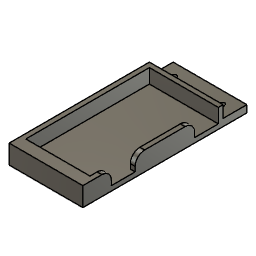
HC-05 mount (Autodesk Fusion 360 design; units mm, degrees)
Autodesk Fusion 360 part; units mm, degrees
sketch "Sketch1" plane through (0, 0, 0) normal (0, 1, 0) x (1, 0, 0)
  line L0 (0, 0) -> (13.5, 0)
  line L1 (13.5, 0) -> (13.5, 27.5)
  line L2 (13.5, 27.5) -> (0, 27.5)
  line L3 (0, 27.5) -> (0, 0)
  dimension "d1" = 13.5
  dimension "d2" = 27.5
  constraint horizontal L0
  constraint vertical L1
  constraint horizontal L2
  constraint vertical L3
  constraint coincident L0.start L3.end
  measures "d1" distance of L0.start L0.end
  measures "d2" distance of L0.start L2.end
extrude "Extrude1" add sketch "Sketch1" along normal blind 1
sketch "Sketch2" plane through (0, 0, 0) normal (0, -1, 0) x (1, 0, 0)
  line L0 (0, 0) -> (0, -27.5)
  line L1 (0, -27.5) -> (13.5, -27.5)
  line L2 (13.5, -27.5) -> (13.5, 0)
  line L3 (13.5, 0) -> (0, 0)
  line L4 (0, -27.5) -> (13.5, -27.5)
  line L5 (13.5, -27.5) -> (13.5, 0)
  line L6 (13.5, 0) -> (0, 0)
  line L7 (0, 0) -> (0, -27.5)
  line L8 (-1, -28.5) -> (14.5, -28.5)
  line L9 (14.5, -28.5) -> (14.5, 1)
  line L10 (14.5, 1) -> (-1, 1)
  line L11 (-1, 1) -> (-1, -28.5)
  dimension "d5" = 1
  constraint horizontal L4
  constraint vertical L5
  constraint horizontal L6
  constraint vertical L7
  constraint coincident L2.end L3.start
  constraint coincident L0.end L1.start
extrude "Extrude2" add sketch "Sketch2" against normal blind 4
sketch "Sketch3" plane through (14.5, 0, 0) normal (1, 0, 0) x (0, 0, -1)
  line L0 (-1, 0) -> (28.5, 0)
  line L1 (28.5, 0) -> (28.5, 4)
  line L2 (28.5, 4) -> (-1, 4)
  line L3 (-1, 4) -> (-1, 0)
  line L4 (28.5, 4) -> (27.5, 4)
  line L5 (27.5, 4) -> (22.5, 4)
  line L6 (22.5, 4) -> (22.5, 1)
  line L7 (22.5, 1) -> (27.5, 1)
  line L8 (27.5, 1) -> (27.5, 4)
  line L9 (-1, 4) -> (5, 4)
  line L10 (5, 4) -> (10, 4)
  line L11 (10, 4) -> (10, 1)
  line L12 (10, 1) -> (5, 1)
  line L13 (5, 1) -> (5, 4)
  dimension "d8" = 5
  dimension "d9" = 6
  dimension "d10" = 5
  dimension "d11" = 3
  constraint coincident L1.end L2.start
  constraint coincident L2 L4.end
  constraint perpendicular L1 L4
  constraint horizontal L5
  constraint vertical L6
  constraint horizontal L7
  constraint vertical L8
  constraint coincident L2.end L3.start
  constraint perpendicular L3 L9
  constraint horizontal L10
  constraint vertical L11
  constraint horizontal L12
  constraint vertical L13
  measures "d8" distance of L4.end L5.end
  measures "d9" distance of L2.end L9.end
  measures "d10" distance of L9.end L10.end
  measures "d11" distance of L9.end L12.end
extrude "Extrude3" cut sketch "Sketch3" against normal blind 1 contours L2 L10 L11 L12 L13 | L2 L5 L6 L7 L8
fillet "Fillet1" radius 2 3 edges at (14, 4, -5) (14, 4, -10) (14, 4, -22.5)
sketch "Sketch4" plane through (0, 0, 0) normal (0, 0, -1) x (-1, 0, 0)
  line L0 (-13.5, 1) -> (0, 1)
  line L1 (0, 1) -> (0, 4)
  line L2 (0, 4) -> (-13.5, 4)
  line L3 (-13.5, 4) -> (-13.5, 1)
  line L4 (-13.5, 4) -> (0, 4)
  line L5 (0, 4) -> (0, 3.5)
  line L6 (0, 3.5) -> (-13.5, 3.5)
  line L7 (-13.5, 3.5) -> (-13.5, 4)
  constraint horizontal L4
  constraint vertical L5
  constraint horizontal L6
  constraint vertical L7
  constraint coincident L1 L5.end
  constraint coincident L2.end L3.start
extrude "Extrude4" add sketch "Sketch4" along normal blind 1.5 contours L1 L2 L3 L4 L5 L6 L7
fillet "Fillet2" radius 1.75 1 edges at (6.75, 3.5, 0)
sketch "Sketch5" plane through (0, 0, -28.5) normal (0, 0, -1) x (-1, 0, 0)
  line L0 (-14.5, 0) -> (1, 0)
  line L1 (1, 0) -> (1, 4)
  line L2 (1, 4) -> (-14.5, 4)
  line L3 (-14.5, 4) -> (-14.5, 0)
  line L4 (-14.5, 0) -> (1, 0)
  line L5 (1, 0) -> (1, 1.5)
  line L6 (1, 1.5) -> (-14.5, 1.5)
  line L7 (-14.5, 1.5) -> (-14.5, 0)
  dimension "d20" = 1.5
  constraint horizontal L4
  constraint vertical L5
  constraint horizontal L6
  constraint vertical L7
  constraint coincident L0.start L3.end
  measures "d20" distance of L0.start L6.end
extrude "Extrude5" add sketch "Sketch5" along normal blind 5 contours L0 L1 L3 L4 L5 L6 L7
sketch "Sketch6" plane through (0, 1.5, 0) normal (0, 1, 0) x (-1, 0, 0)
  line L0 (1, -28.5) -> (-14.5, -28.5)
  line L1 (-14.5, -28.5) -> (-14.5, -33.5)
  line L2 (-14.5, -33.5) -> (1, -33.5)
  line L3 (1, -33.5) -> (1, -28.5)
  point P0 (-11.83, -31)
  point P1 (-1.67, -31)
  dimension "d23" = 10.16
  dimension "d24" = 2.67
  dimension "d29" = 2.5
  measures "d23" distance of P0 P1
  measures "d24" distance of L1 P0
  measures "d29" distance of L0 P0
hole "Hole1" at (11.83, 1.5, -31) at (1.67, 1.5, -31) direction (0, -1, 0) diameter 1 depth 4 tip angle 118
